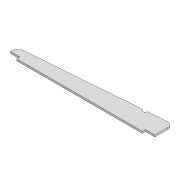
# Autodesk Inventor part: rail
Saved by Autodesk Inventor 2020 (Build 240168000, 168)
## iProperties
Created: 2021-06-07
Part Number: rail
Material: Generic
Document SubType Name: Modeling
Designer: Aidan Lee
Density: 1 g/cm^3
Appearance: Default
Author: Aidan Lee
Autodesk Inventor part; units mm, degrees
ref_plane "YZ Plane" through (0, 0, 0) normal (1, 0, 0) x (0, 1, 0)
ref_plane "XZ Plane" through (0, 0, 0) normal (0, 1, 0) x (-1, 0, 0)
ref_plane "XY Plane" through (0, 0, 0) normal (0, 0, 1) x (1, 0, 0)
sketch "Sketch2" plane through (0, 0, 0) normal (0, 1, 0) x (-1, 0, 0)
  line L0 (0, 0) -> (-228, 0)
  line L1 (-228, 0) -> (-228, -33.6943)
  line L2 (-228, -33.6943) -> (0, -16)
  arc A0 (-228, -25.5205) -> (-219.8507, -33.0618) centre (-220.436, -25.5205) ccw
  arc A1 (-184.5652, -29.4637) -> (-190.2978, -29.9086) centre (-187.3652, -30.5408) ccw
  arc A2 (-191.378, -30.8522) -> (-190.2978, -29.9086) centre (-191.4709, -29.6558) ccw
  arc A3 (-184.5652, -29.4637) -> (-183.3523, -30.2293) centre (-183.4452, -29.0329) ccw
  line L3 (0, 0) -> (-15, 0)
  line L4 (-15, 0) -> (-15, -5)
  line L5 (-15, -5) -> (0, -5)
  line L6 (-228, 0) -> (-213, 0)
  line L7 (-213, 0) -> (-213, -5)
  line L8 (-213, -5) -> (-228, -5)
  line L9 (-228, -5) -> (-228, 0)
  line L10 (0, -16) -> (0, -5)
  arc A4 (-9.97, -16.7737) -> (0, -6) centre (-10.8061, -6) ccw
  point P0 (-220.5, -5)
  point P1 (-7.5, -5)
  point P2 (-15, 0)
  dimension "xp" = 228
  dimension "corner" = 7.564
  dimension "d9" = 1.2
  dimension "d10" = 1.2
  dimension "d15" = 15
  dimension "d16" = 3
  dimension "d20" = 15
  dimension "cutoutdepth" = 5
  dimension "cutoutlength" = 198
  dimension "theta" = 4.438
  dimension "raised" = 11
  dimension "d25" = 10.8061
  dimension "d26" = 1
  constraints: 22 end point, 12 point on circle, 8 tangent, 7 point on line, 5 centre point, 3 horizontal, 3 parallel, 3 perpendicular, 2 midpoint, 1 horizontal alignment, 1 vertical
  measures "xp" distance of L0.start L0.end
  measures "corner" radius of A0
  measures "d9" radius of A2
  measures "d10" radius of A3
  measures "d15" distance between parallel lines of L1 L7
  measures "d16" radius of A1
  measures "d20" distance between parallel lines of L10 L4
  measures "cutoutdepth" distance between parallel lines of L0 L5
  measures "cutoutlength" distance between parallel lines of L7 L4
  measures "theta" angle of L2 L0
  measures "raised" distance from line of L2.end L5
  measures "d25" radius of A4
  measures "d26" distance from line of L5 A4.end
extrude "Extrusion1" add sketch "Sketch2" along normal blind 3 contours L4 L5 L10 A4 L2 A3 A1 A2 A0 L1 L8 L7 L0
equation "\"d15\" = cutoutoffset"
equation "\"d20\" = cutoutoffset"
equation "\"b\" = 17.7"
equation "\"cutoutoffset\" = 15"
body "Solid1"
